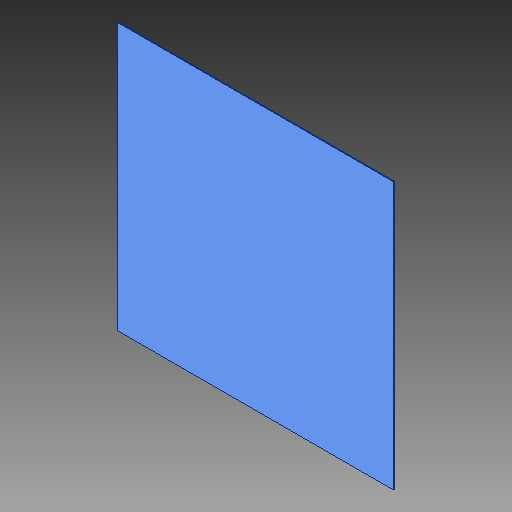
# Autodesk Inventor part: 2_2UH
Saved by Autodesk Inventor 2018 (Build 220112000, 112)
## iProperties
Created: 2015-11-24
Part Number: 2_2UH
Material: Generic
Document SubType Name: Modeling
Designer: PhillipD
Density: 1 g/cm^3
Appearance: L-NR3010, 2_2UH
Author: PhillipD
Autodesk Inventor part; units mm, degrees
ref_plane "YZ Plane" through (0, 0, 0) normal (1, 0, 0) x (0, 1, 0)
ref_plane "XZ Plane" through (0, 0, 0) normal (0, 1, 0) x (-1, 0, 0)
ref_plane "XY Plane" through (0, 0, 0) normal (0, 0, 1) x (1, 0, 0)
sketch "L-NR3010, 2_2UH_81" plane through (0, 0, 0) normal (0, 0, 1) x (1, 0, 0)
  line L0 (-1.6, 1.6) -> (1.6, 1.6)
  line L1 (1.6, 1.6) -> (1.6, -1.5)
  line L2 (1.6, -1.5) -> (-1.6, -1.5)
  line L3 (-1.6, -1.5) -> (-1.6, 1.6)
  constraints: 8 end point
extrude "Extrusion1" add sketch "L-NR3010, 2_2UH_81" along normal blind 0.01
body "Solid1"
